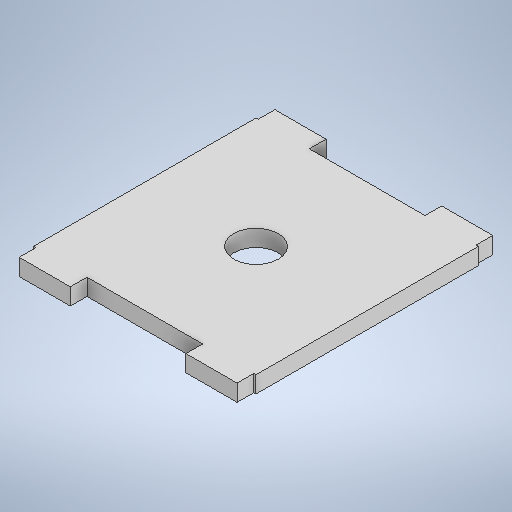
# Autodesk Inventor part: A_beam_end_mound_1
Saved by Autodesk Inventor 2025.2 (Build 292293000, 293)
## iProperties
Created: 2025-05-02
Part Number: A_beam_end_mound_1
Material: Generic
Document SubType Name: Sheet Metal
Designer: Caspe
Density: 1 g/cm^3
Sheet Metal Rule: Default_mm
Appearance: Default
Author: Caspe
Autodesk Inventor part; units mm, degrees
ref_plane "YZ Plane" through (0, 0, 0) normal (1, 0, 0) x (0, 1, 0)
ref_plane "XZ Plane" through (0, 0, 0) normal (0, 1, 0) x (-1, 0, 0)
ref_plane "XY Plane" through (0, 0, 0) normal (0, 0, 1) x (1, 0, 0)
sketch "Sketch1" plane through (0, 0, 0) normal (0, 1, 0) x (-1, 0, 0)
  line L0 (0, 0) -> (40, 0)
  line L1 (40, 0) -> (40, -40)
  line L2 (40, -40) -> (0, -40)
  line L3 (0, -40) -> (0, 0)
  line L4 (0, 0) -> (9.6, 0)
  line L5 (9.6, 0) -> (9.6, 3)
  line L6 (9.6, 3) -> (0.4, 3)
  line L7 (0.4, 3) -> (0.4, 0)
  line L8 (40, -20) -> (0, -20)
  line L9 (20, 0) -> (20, -40)
  circle A0 centre (20, -20) radius 4
  line L10 (30.4, 0) -> (30.4, 3)
  line L11 (30.4, 3) -> (39.6, 3)
  line L12 (39.6, 3) -> (39.6, 0)
  line L13 (9.6, -40) -> (9.6, -43)
  line L14 (9.6, -43) -> (0.4, -43)
  line L15 (0.4, -43) -> (0.4, -40)
  line L16 (30.4, -40) -> (30.4, -43)
  line L17 (30.4, -43) -> (39.6, -43)
  line L18 (39.6, -43) -> (39.6, -40)
  point P0 (9.6, 0)
  dimension "d0" = 40
  dimension "d1" = 40
  dimension "d2" = 9.2
  dimension "d3" = 3
  dimension "d5" = 8
  dimension "d6" = 0.4
  measures "d0" distance of L1.end L2.end
  measures "d1" distance of L0.end L1.end
  measures "d2" distance of L6.end L5.end
  measures "d3" distance of L5.end L4.end
  measures "d5" diameter of A0
  measures "d6" distance between parallel lines of L3 L7
extrude "Plate1" add sketch "Sketch1" along normal blind 3 contours L0 L9 A0 L8 L3 | L7 L6 L5 L0 | L8 A0 L9 L2 L3 | L0 L1 L8 A0 L9 | L2 L13 L14 L15 | A0 L8 L1 L2 L9 | L10 L11 L12 L0 | L2 L18 L17 L16
equation "\"d4\" = Thickness"
equation "\"BendRadius\" = Thickness"
equation "\"BendReliefWidth\" = Thickness"
equation "\"BendReliefDepth\" = 0.5 * Thickness"
equation "\"CornerReliefSize\" = 4 * Thickness"
equation "\"MinimumRemnant\" = 2 * Thickness"
equation "\"TransitionRadius\" = BendRadius"
equation "\"JacobiRadiusSize\" = BendRadius"
equation "\"GapSize\" = Thickness"
equation "\"Thickness\" = 3"
body "Solid1"
